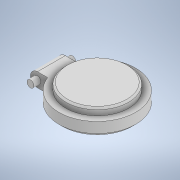
# Autodesk Inventor part: Access Hatch
Saved by Autodesk Inventor 2022 (Build 260153000, 153)
## iProperties
Created: 2021-10-22
Part Number: Access Hatch
Material: Generic
Document SubType Name: Modeling
Designer: tgr41
Density: 1 g/cm^3
Appearance: Default
Author: tgr41
Autodesk Inventor part; units mm, degrees
ref_plane "YZ Plane" through (0, 0, 0) normal (1, 0, 0) x (0, 1, 0)
ref_plane "XZ Plane" through (0, 0, 0) normal (0, 1, 0) x (-1, 0, 0)
ref_plane "XY Plane" through (0, 0, 0) normal (0, 0, 1) x (1, 0, 0)
sketch "Sketch1" plane through (0, 0, 0) normal (0, 1, 0) x (-1, 0, 0)
  circle A0 centre (110.109, -133.985) radius 57.15
  circle A1 centre (110.109, -133.985) radius 50.8
  circle A2 centre (110.109, -133.985) radius 69.85
  line L0 (206.4385, -159.385) -> (175.1771, -159.385)
  line L1 (206.4385, -159.385) -> (206.4385, -108.585)
  line L2 (206.4385, -108.585) -> (175.1771, -108.585)
  point P0 (0, 0)
  dimension "d51" = 139.7
  dimension "d11" = 114.3
  dimension "d12" = 101.6
  constraints: 6 end point, 2 centre point, 2 coincident, 3 other
  measures "d11" diameter of A0
  measures "d12" diameter of A1
extrude "Extrusion11" add sketch "Sketch1" against normal blind 25.4 contours A0 | A1 | A2 | A2 L2 L1 L0
extrude "Extrusion12" add sketch "Sketch1" along normal blind 12.7 contours A0 | A1
chamfer "Chamfer1" distance 3.175 angle 45 1 edges at (-52.959, 12.7, -133.985)
chamfer "Chamfer2" distance 6.35 angle 45 1 edges at (-40.259, -25.4, -133.985)
fillet "Fillet2" radius 12.7 2 edges at (-206.4385, -25.4, -133.985) (-206.4385, 0, -133.985)
sketch "Sketch5" plane through (-175.1771, -19.05, -108.585) normal (0, 0, 1) x (1, 0, 0)
  arc A0 (-18.5614, 19.05) -> (-18.5614, -6.35) centre (-18.5614, 6.35) ccw projected
  circle A1 centre (-18.5614, 6.35) radius 6.35
  point P0 (175.1771, 19.05)
  dimension "d63" = 12.7
  constraints: 1 centre point, 1 coincident
  measures "d63" diameter of A1
extrude "Extrusion13" add sketch "Sketch5" along normal blind 12.7
sketch "Sketch6" plane through (-175.1771, -19.05, -159.385) normal (0, 0, -1) x (-1, 0, 0)
  arc A0 (18.5614, -6.35) -> (18.5614, 19.05) centre (18.5614, 6.35) ccw projected
  circle A1 centre (18.5614, 6.35) radius 6.35
  point P0 (-175.1771, 19.05)
  dimension "d66" = 12.7
  constraints: 1 centre point, 1 coincident
  measures "d66" diameter of A1
extrude "Extrusion14" add sketch "Sketch6" along normal blind 12.7
body "Solid3"
